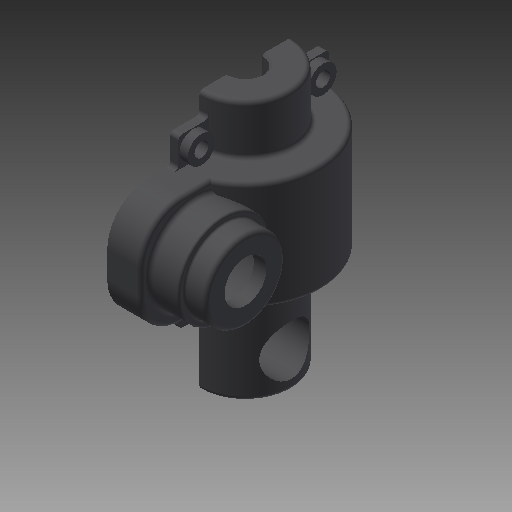
# Autodesk Inventor part: 400-01
Saved by Autodesk Inventor 2019 (Build 230136000, 136)
## iProperties
Company: Autodesk Inc.
Created: 2007-11-20
Part Number: 400-01
Document SubType Name: Modeling
Designer: Autodesk Inc.
Density: 1.06 g/cm^3
Mass: 15.4397 g
Surface Area: 94.4346 cm^2
Volume: 14.5658 cm^3
Material: ABS Plastic
Description: GEAR  HOUSING CASE L
Appearance: Gray
Component Category: Lower Component
Author: Inventor
Autodesk Inventor part; units mm, degrees
ref_plane "YZ Plane" through (0, 0, 0) normal (1, 0, 0) x (0, 1, 0)
ref_plane "XZ Plane" through (0, 0, 0) normal (0, 1, 0) x (-1, 0, 0)
ref_plane "XY Plane" through (0, 0, 0) normal (0, 0, 1) x (1, 0, 0)
sketch "Sketch1" plane through (0, 0, 0) normal (0, 1, 0) x (-1, 0, 0)
  circle A0 centre (0, 0) radius 11
  dimension "d0" = 22
  constraints: 1 centre point, 1 coincident
  measures "d0" diameter of A0
extrude "Extrusion1" add sketch "Sketch1" along normal blind 62
ref_plane "Work Plane1" through (0, 24, 0) normal (0, -1, 0) x (1, 0, 0)
sketch "Sketch2" plane through (0, 24, 0) normal (0, -1, 0) x (1, 0, 0)
  circle A0 centre (0, 0) radius 11 projected
  circle A1 centre (0, 0) radius 18
  dimension "d4" = 36
  constraints: 1 centre point, 1 coincident
  measures "d4" diameter of A1
extrude "Extrusion2" add sketch "Sketch2" against normal blind 26
sketch "Sketch3" plane through (0, 0, 0) normal (1, 0, 0) x (0, 1, 0)
  line L0 (50, -18) -> (24, -18) projected
  line L1 (24, -18) -> (24, -11) projected
  line L2 (24, -11) -> (0, -11) projected
  line L3 (0, -11) -> (0, 11) projected
  line L4 (0, 11) -> (24, 11) projected
  line L5 (24, 11) -> (24, 18) projected
  line L6 (24, 18) -> (50, 18) projected
  line L7 (50, 18) -> (50, 11) projected
  line L8 (50, 11) -> (62, 11) projected
  line L9 (62, 11) -> (62, -11) projected
  line L10 (62, -11) -> (50, -11) projected
  line L11 (50, -11) -> (50, -18) projected
  circle A0 centre (37, 20) radius 11
  line L12 (0, 0) -> (62, 0) construction
  line L13 (24, 18) -> (50, 18)
  line L14 (50, 18) -> (50, 33)
  line L15 (50, 33) -> (24, 33)
  line L16 (24, 33) -> (24, 18)
  line L17 (24, 18) -> (50, 18)
  line L18 (50, 18) -> (50, 14.5)
  line L19 (50, 14.5) -> (24, 14.5)
  line L20 (24, 14.5) -> (24, 18)
  circle A1 centre (37, 20) radius 9.5
  circle A2 centre (37, 20) radius 8.5
  line L21 (56, 9.05) -> (41.5, 9.05)
  line L22 (17.85, 9.05) -> (17.85, 0)
  line L23 (62, 4.05) -> (56, 4.05)
  line L24 (56, 4.05) -> (56, 9.05)
  line L25 (32.5, 9.05) -> (17.85, 9.05)
  line L26 (41.5, 9.05) -> (41.5, 16)
  line L27 (32.5, 16) -> (41.5, 16)
  line L28 (32.5, 16) -> (32.5, 9.05)
  line L29 (17.85, 0) -> (62, 0)
  line L30 (62, 0) -> (62, 4.05)
  circle A3 centre (8.3747, 0) radius 6
  point P0 (37, 33)
  point P1 (37, 16)
  point P2 (37.6253, 20)
  dimension "d7" = 22
  dimension "d8" = 20
  dimension "d9" = 15
  dimension "d10" = 13
  dimension "d15" = 19
  dimension "d16" = 17
  dimension "d25" = 9.05
  dimension "d26" = 9
  dimension "d28" = 6
  dimension "d29" = 4.05
  dimension "d30" = 2
  dimension "d31" = 14.65
  dimension "d34" = 12
  dimension "d35" = 8.3747
  dimension "d67" = 26
  dimension "d99" = 0.6253
  constraints: 38 end point, 5 midpoint, 5 parallel, 4 centre point, 4 perpendicular, 4 point on line, 2 coincident, 2 collinear, 2 horizontal, 1 vertical alignment, 1 other
  measures "d7" diameter of A0
  measures "d8" distance from line of A0.centre L12
  measures "d9" distance of L13.end L14.end
  measures "d10" distance from line of A0.centre L5
  measures "d15" diameter of A1
  measures "d16" diameter of A2
  measures "d25" distance of L22.start L22.end
  measures "d26" distance between parallel lines of L26 L28
  measures "d28" distance between parallel lines of L9 L24
  measures "d29" distance between parallel lines of L29 L23
  measures "d30" distance between parallel lines of L6 L27
  measures "d31" distance between parallel lines of L28 L22
  measures "d34" diameter of A3
  measures "d35" distance from line of L3 A3.centre
  measures "d67" distance of L14.end L15.end
  measures "d99" distance of point (37.625, 20) A0.centre
extrude "Extrusion3" add sketch "Sketch3" against normal mid plane 16 contours L5 L6 A0 L19 | L16 L15 L14 L6 A0 | A0 L6 A1 L19 | L19 A0 L6 L7 | A0 L6 A1 | A1 L6 A2 L19 | L19 A1 L6 A0 | A1 L6 A2 | A2 L6 L19 L26 L27 L28 | L19 A2 L6 A1 | A2 L6 | L28 L27 L26 L19
extrude "Extrusion4" add sketch "Sketch3" along normal mid plane 30 contours L19 A1 L28 A0 | A0 L6 A1 L19 | L28 A1 L26 A0 | A0 L6 A1 | A1 L6 A2 L19 | L19 A2 L28 A1 | L19 A1 L6 A0 | A0 L26 A1 L19 | L28 A2 L26 A1 | A1 L6 A2 | A2 L6 L19 L26 L27 L28 | L19 L28 A2 | A1 L26 A2 L19 | L19 A2 L6 A1 | L28 L19 L26 A2 | A2 L6 | L28 L27 L26 L19 | A2 L26 L19
extrude "Extrusion5" add sketch "Sketch3" against normal mid plane 40 contours A1 L6 A2 L19 | L19 A2 L28 A1 | L28 A2 L26 A1 | A1 L6 A2 | A2 L6 L19 L26 L27 L28 | L19 L28 A2 | A1 L26 A2 L19 | L19 A2 L6 A1 | L28 L19 L26 A2 | A2 L6 | L28 L27 L26 L19 | A2 L26 L19
extrude "Extrusion6" cut sketch "Sketch3" along normal mid plane 34 contours A2 L6 L19 L26 L27 L28 | L19 L28 A2 | L28 L19 L26 A2 | A2 L6 | L28 L27 L26 L19 | A2 L26 L19
revolve "Revolution1" cut sketch "Sketch3" angle 360 about axis through (0, 0, 0) along (0, 1, 0) contours L29 L22 L25 L28 A0 L26 L21 L24 L23 L9 | L28 A1 L26 A0 | L28 A2 L26 A1 | L28 L19 L26 A2 | L28 L27 L26 L19
split "Split1" plane through (0, 0, 0) removes the side toward (1, 0, 0)
extrude "Extrusion7" cut sketch "Sketch3" along normal through all both and the other way through all contours A3
sketch "Sketch4" plane through (-20, 37, 20) normal (-1, 0, 0) x (0, 0, 1)
  circle A0 centre (0, 0) radius 9.5 projected
  circle A1 centre (0, 0) radius 5
  dimension "d40" = 10
  constraints: 1 centre point, 1 coincident
  measures "d40" diameter of A1
extrude "Extrusion8" cut sketch "Sketch4" against normal through all contours A1
fillet "Fillet7" radius 10 2 edges at (-4, 24, 33) (-4, 50, 33)
fillet "Fillet8" radius 1 7 edges at (-8, 24, 19.5623) (-8, 26.9289, 30.0711) (-8, 37, 33) (-8, 47.0711, 30.0711) (-8, 50, 19.5623) (-8, 37, 31) (-20, 27.5, 20)
fillet "Fillet9" radius 0.5 2 edges at (-15, 37, 31) (-15, 27.5, 20)
sketch "Sketch5" plane through (0, 37, 20) normal (1, 0, 0) x (0, 0, -1)
  circle A0 centre (20, -28.6253) radius 6 projected
  line L0 (9, -13) -> (-3, -13) projected
  line L1 (9, -13) -> (2, -13)
  line L2 (2, -13) -> (2, -20)
  line L3 (2, -20) -> (9, -20)
  line L4 (9, -20) -> (9, -13)
  line L5 (9, -20) -> (11, -20)
  line L6 (11, -20) -> (11, -13)
  line L7 (11, -13) -> (9, -13)
  line L8 (9, -13) -> (9, -20)
  line L9 (-13, -3) -> (-13, 3) projected
  line L10 (-3, 13) -> (9, 13) projected
  line L11 (-13, 0) -> (-30.6999, 0) construction
  line L12 (20, -28.6253) -> (20, -23.9824) construction
  line L13 (9, 13) -> (2, 13)
  line L14 (2, 13) -> (2, 20)
  line L15 (2, 20) -> (9, 20)
  line L16 (9, 20) -> (9, 13)
  line L17 (9, 20) -> (11, 20)
  line L18 (11, 20) -> (11, 13)
  line L19 (11, 13) -> (9, 13)
  line L20 (9, 13) -> (9, 20)
  line L21 (31, -13) -> (38, -13)
  line L22 (38, -13) -> (38, -20)
  line L23 (38, -20) -> (31, -20)
  line L24 (31, -20) -> (31, -13)
  line L25 (31, -20) -> (29, -20)
  line L26 (29, -20) -> (29, -13)
  line L27 (29, -13) -> (31, -13)
  line L28 (31, -13) -> (31, -20)
  line L29 (31, 13) -> (38, 13)
  line L30 (38, 13) -> (38, 20)
  line L31 (38, 20) -> (31, 20)
  line L32 (31, 20) -> (31, 13)
  line L33 (29, 13) -> (31, 13)
  line L34 (31, 20) -> (29, 20)
  line L35 (29, 20) -> (29, 13)
  line L36 (31, 13) -> (31, 20)
  circle A1 centre (34.5, -16.5) radius 3.25
  circle A2 centre (34.5, 16.5) radius 3.25
  circle A3 centre (5.5, 16.5) radius 3.25
  circle A4 centre (5.5, -16.5) radius 3.25
  point P0 (31, 23)
  point P1 (-8.5, 0)
  point P2 (31, 13)
  dimension "d51" = 7
  dimension "d52" = 7
  dimension "d53" = 3.5
  dimension "d54" = 3.5
  dimension "d78" = 6.5
  dimension "d79" = 6.5
  dimension "d80" = 6.5
  dimension "d81" = 6.5
  dimension "d91" = 2
  constraints: 68 end point, 25 symmetric about line, 5 parallel, 4 centre point, 4 coincident, 3 perpendicular, 2 horizontal, 1 midpoint, 1 point on line
  measures "d51" distance between parallel lines of L1 L3
  measures "d52" distance of L2.end L3.end
  measures "d53" distance from line of L3 point (5.5, -16.5)
  measures "d54" distance from line of L2 point (5.5, -16.5)
  measures "d78" diameter of A1
  measures "d79" diameter of A2
  measures "d80" diameter of A3
  measures "d81" diameter of A4
  measures "d91" distance between parallel lines of L8 L6
extrude "Extrusion9" add sketch "Sketch5" against normal blind 2 contours L4 L3 L2 L0 | L7 L6 L5 L4 | L14 L15 L16 L10 | L16 L17 L18 L19 | L21 L22 L23 L24 | L24 L25 L26 L27 | L32 L31 L30 L29 | L33 L35 L34 L32 | A1 | A2 | A3 | A4
extrude "Extrusion11" add sketch "Sketch5" against normal blind 4 contours A1 | A2 | A3 | A4
hole "Hole2" at (0, 53.5, -14.5) at (0, 20.5, -14.5) at (0, 20.5, 14.5) at (0, 53.5, 14.5) direction (-1, 0, 0) diameter 3.4 end through all clearance for "Countersunk Flat Head Screw ISO 2009/7046" size "M3" standard "ISO"
chamfer "Chamfer1" distance 0.5 angle 45 2 edges at (-4.05, 56, 0) (-4.05, 62, 0)
fillet "Fillet13" radius 1 6 edges at (-11, 62, 0) (-17.8136, 50, -2.5839) (-17.8136, 24, -2.5839) (-11, 24, 0) (-11, 0, 0) (-11, 50, 0)
fillet "Fillet14" radius 1 6 edges at (-1, 57, 18) (-1.0042, 57, 10.9541) (-1, 50, 18) (-1, 17, 18) (-1.0042, 17, 10.9541) (-1, 24, 18)
fillet "Fillet15" radius 1 4 edges at (-1, 57, -18) (-1.0042, 57, -10.9541) (-1, 17, -18) (-1.0042, 17, -10.9541)
mirror "Mirror1" about plane through (0, 0, 0) normal (1, 0, 0) remove original yes
equation "\"d51\" = d52"
equation "\"d53\" = 0.5 * d51"
equation "\"d54\" = 0.5 * d52"
equation "\"d79\" = d78"
equation "\"d80\" = d78"
equation "\"d81\" = d78"
body "Solid1"
